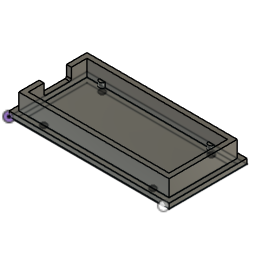
bottom (Autodesk Fusion 360 design; units mm, degrees)
Autodesk Fusion 360 part; units mm, degrees
note: some values were not read from the file. Set by a fixed rule: which sketch regions a step uses.
sketch "Skizze1" plane through (0, 0, 0) normal (0, 0, 1) x (1, 0, 0)
  line L0 (0, 0) -> (52.6, 0)
  line L1 (52.6, 0) -> (52.6, 25.6)
  line L2 (52.6, 25.6) -> (0, 25.6)
  line L3 (0, 25.6) -> (0, 0)
  line L4 (0, 0) -> (50.8, 0)
  line L5 (3.2, 3.2) -> (49.4, 3.2)
  line L6 (49.4, 3.2) -> (49.4, 22.4)
  line L7 (49.4, 22.4) -> (3.2, 22.4)
  line L8 (3.2, 22.4) -> (3.2, 3.2)
  line L9 (1.6, 24) -> (51, 24)
  line L10 (51, 24) -> (51, 1.6)
  line L11 (51, 1.6) -> (1.6, 1.6)
  line L12 (1.6, 1.6) -> (1.6, 24)
  circle A0 centre (8.2, 22.4) radius 1
  circle A1 centre (44.1, 22.4) radius 1
  circle A2 centre (44.1, 3.2) radius 1
  circle A3 centre (8.2, 3.2) radius 1
  dimension "d2" = 46.2
  dimension "d3" = 19.2
  dimension "d4" = 1.6
  dimension "d6" = 1.6
  dimension "d7" = 1.6
  dimension "d8" = 1.6
  dimension "d13" = 1.6
  dimension "d14" = 1.6
  dimension "d15" = 1.6
  dimension "d16" = 1.6
  dimension "d28" = 2
  dimension "d29" = 2
  dimension "d30" = 2
  dimension "d31" = 2
  dimension "d32" = 5.3
  dimension "d33" = 5.3
  dimension "d34" = 5
  dimension "d35" = 5
  constraint horizontal L0
  constraint vertical L1
  constraint horizontal L2
  constraint vertical L3
  constraint coincident L0.start L3.end
  constraint horizontal L4
  constraint horizontal L5
  constraint vertical L6
  constraint horizontal L7
  constraint vertical L8
  constraint horizontal L9
  constraint vertical L10
  constraint horizontal L11
  constraint vertical L12
  constraint coincident L7 A0.centre
  constraint coincident L7 A1.centre
  constraint coincident L5 A3.centre
  constraint coincident L5 A2.centre
  measures "d2" distance of L5.start L5.end
  measures "d3" distance of L5.end L6.end
  measures "d4" distance of L5 L11
  measures "d6" distance of L0 L11
  measures "d7" distance of L8 L12
  measures "d8" distance of L3 L12
  measures "d13" distance of L6 L10
  measures "d14" distance of L1 L10
  measures "d15" distance of L7 L9
  measures "d16" distance of L2 L9
  measures "d28" diameter of A0
  measures "d29" diameter of A1
  measures "d30" diameter of A2
  measures "d31" diameter of A3
  measures "d32" distance of L6.end A1.centre
  measures "d33" distance of L6 A2.centre
  measures "d34" distance of L7.end A0.centre
  measures "d35" distance of L5.start A3.centre
extrude "Extrusion1" add sketch "Skizze1" along normal blind 1.6 contours L0 L1 L2 L3 L4 | L5 L6 L7 L8 A0 A1 A2 A3 | L5 A2 | L5 A2 | L5 A3 | L5 A3 | L7 A1 | L7 A1 | L7 A0 | L7 A0 | L9 L10 L11 L12
extrude "Extrusion2" add sketch "Skizze1" along normal blind 7 contours L5 A2 | L5 A3 | L7 A1 | L7 A0 | L9 L10 L11 L12 picked at (44.1779, 2.8253) picked at (7.9246, 2.9129) picked at (44.3078, 22.76) picked at (8.5222, 22.5479)
ref_plane "Arbeitsebene1" through (1.6, 12.8, 4.3) normal (-1, 0, 0) x (0, -1, 0)
sketch "Skizze2" plane through (1.6, 0, 0) normal (-1, 0, 0) x (0, -1, 0)
  line L0 (-17.3, 7) -> (-8.3, 7)
  line L1 (-8.3, 7) -> (-8.3, 3.7)
  line L2 (-8.8, 3.2) -> (-16.8, 3.2)
  line L3 (-17.3, 3.7) -> (-17.3, 7)
  line L4 (-24, 7) -> (-1.6, 7)
  line L5 (-25.6, 1.6) -> (0, 1.6)
  arc A0 (-17.3, 3.7) -> (-16.8, 3.2) centre (-16.8, 3.7) ccw
  arc A1 (-8.8, 3.2) -> (-8.3, 3.7) centre (-8.8, 3.7) ccw
  dimension "d22" = 1.6
  dimension "d23" = 9
  dimension "d24" = 0.5
  dimension "d25" = 0.5
  constraint horizontal L0
  constraint vertical L1
  constraint horizontal L2
  constraint vertical L3
  constraint coincident L0.start L4
  constraint midpoint L0 L4
  constraint tangent L3 A0
  constraint tangent L2 A0
  constraint tangent L2 A1
  constraint tangent L1 A1
  measures "d22" distance of L2 L5
  measures "d23" distance of L1 L3
  measures "d24" radius of A0
  measures "d25" radius of A1
extrude "Extrusion3" cut sketch "Skizze2" against normal blind 1.6
extrude "Extrusion4" add sketch "Skizze1" along normal blind 3.2 contours L5 A2 | L5 A3 | L7 A1 | L7 A0 picked at (44.0258, 3.6243) picked at (8.0222, 3.8816) picked at (44.3444, 22.0739) picked at (7.9673, 21.807)
equation "d19 = 1.6 mm + 4.9 mm + 0.5 mm"
